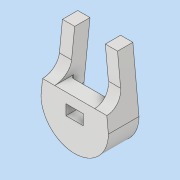
# Autodesk Inventor part: servoPotentiometerAttachment
Saved by Autodesk Inventor 2017 (Build 210142000, 142)
## iProperties
Created: 2016-12-10
Part Number: servoPotentiometerAttachment
Material: ABS Plastic
Document SubType Name: Modeling
Designer: techn
Density: 1.06 g/cm^3
Appearance: Smooth - White
Author: techn
Autodesk Inventor part; units mm, degrees
ref_plane "YZ Plane" through (0, 0, 0) normal (1, 0, 0) x (0, 1, 0)
ref_plane "XZ Plane" through (0, 0, 0) normal (0, 1, 0) x (-1, 0, 0)
ref_plane "XY Plane" through (0, 0, 0) normal (0, 0, 1) x (1, 0, 0)
sketch "Sketch1" plane through (0, 0, 0) normal (0, 0, 1) x (1, 0, 0)
  circle A0 centre (0, 0) radius 4.445
  line L0 (0, 0) -> (0, 12.7)
  line L1 (0, 12.7) -> (-3.175, 12.7)
  line L2 (-3.175, 12.7) -> (3.175, 12.7)
  line L3 (-3.175, 12.7) -> (-4.4221, 0.4502)
  line L4 (3.175, 12.7) -> (4.4221, 0.4502)
  line L5 (-3.175, 12.7) -> (-5.715, 12.7)
  line L6 (-5.715, 12.7) -> (-6.985, 0)
  line L7 (-6.985, 0) -> (-4.445, 0)
  line L8 (3.175, 12.7) -> (5.715, 12.7)
  line L9 (5.715, 12.7) -> (6.985, 0)
  line L10 (6.985, 0) -> (4.445, 0)
  arc A1 (-6.985, 0) -> (6.985, 0) centre (0, 0) ccw
  dimension "d0" = 8.89
  dimension "d1" = 12.7
  dimension "d2" = 3.175
  dimension "d3" = 6.35
  dimension "d4" = 2.54
  dimension "d5" = 2.54
  dimension "d6" = 2.54
  dimension "d7" = 2.54
  constraints: 22 end point, 6 point on circle, 3 horizontal, 2 centre point, 2 parallel, 2 tangent, 1 coincident, 1 concentric, 1 point on line, 1 vertical
  measures "d0" diameter of A0
  measures "d1" distance of L0.start L0.end
  measures "d2" distance of L0.end L1.end
  measures "d3" distance of L1.end L2.end
  measures "d4" distance of L1.end L5.end
  measures "d5" distance of L6.end L7.end
  measures "d6" distance of L2.end L8.end
  measures "d7" distance of L9.end L10.end
extrude "Extrusion1" add sketch "Sketch1" along normal blind 3.175 contours L10 A1 L7 A0 | A0 L4 L8 L9 L10 | L7 L6 L5 L3 A0
sketch "Sketch2" plane through (0, 0, 3.175) normal (0, 0, 1) x (1, 0, 0)
  line L0 (-3.175, 12.7) -> (-5.715, 12.7) projected
  line L1 (-5.715, 12.7) -> (-6.985, 0) projected
  arc A0 (-6.985, 0) -> (6.985, 0) centre (0, 0) ccw projected
  line L2 (6.985, 0) -> (5.715, 12.7) projected
  line L3 (5.715, 12.7) -> (3.175, 12.7) projected
  line L4 (3.175, 12.7) -> (4.4221, 0.4502) projected
  arc A1 (-4.4221, 0.4502) -> (4.4221, 0.4502) centre (0, 0) ccw projected
  line L5 (-4.4221, 0.4502) -> (-3.175, 12.7) projected
  line L6 (-6.6675, 3.175) -> (6.6675, 3.175)
  dimension "d18" = 3.175
  constraints: 2 end point, 2 point on line, 1 horizontal
  measures "d18" distance from line of point (0, 0) L6
ref_plane "Work Plane1" through (0, 0, 6.35) normal (0, 0, 1) x (1, 0, 0)
extrude "Extrusion4" add sketch "Sketch2" along normal blind 3.175 contours L6 L4 A1 L5 | L5 A1 L4 L6 L2 A0 L1
sketch "Sketch4" plane through (0, 0, 6.35) normal (0, 0, 1) x (1, 0, 0)
  line L0 (-1.8034, 1.0795) -> (1.8034, 1.0795)
  line L1 (1.8034, 1.0795) -> (1.8034, -1.0795)
  line L2 (1.8034, -1.0795) -> (-1.8034, -1.0795)
  line L3 (-1.8034, -1.0795) -> (-1.8034, 1.0795)
  point P0 (0, 0)
  dimension "d23" = 3.6068
  dimension "d24" = 2.159
  dimension "d25" = 1.8034
  dimension "d26" = 1.0795
  constraints: 8 end point, 2 parallel, 1 horizontal, 1 perpendicular
  measures "d23" distance of L1.end L2.end
  measures "d24" distance of L0.end L1.end
  measures "d25" distance from line of L1 point (0, 0)
  measures "d26" distance from line of L2 point (0, 0)
extrude "Extrusion6" cut sketch "Sketch4" against normal blind 3.175
fillet "Fillet1" radius 3.175 2 edges at (-5.4061, 3.175, 3.175) (5.4061, 3.175, 3.175)
fillet "Fillet2" radius 0.762 3 edges at (-4.2834, 1.8126, 3.175) (4.2834, 1.8126, 3.175) (0, -4.445, 3.175)
equation "\"d25\" = 0.5 * d23"
equation "\"d26\" = 0.5 * d24"
body "Solid1"
